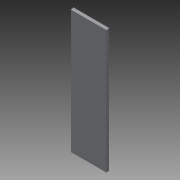
# Autodesk Inventor part: topback
Saved by Autodesk Inventor 2015 (Build 190159000, 159)
## iProperties
Created: 2015-02-03
Part Number: topback
Material: Generic
Document SubType Name: Modeling
Designer: rubidium
Density: 1 g/cm^3
Appearance: Default
Author: rubidium
Autodesk Inventor part; units mm, degrees
ref_plane "YZ Plane" through (0, 0, 0) normal (1, 0, 0) x (0, 1, 0)
ref_plane "XZ Plane" through (0, 0, 0) normal (0, 1, 0) x (-1, 0, 0)
ref_plane "XY Plane" through (0, 0, 0) normal (0, 0, 1) x (1, 0, 0)
sketch "Sketch1" plane through (0, 0, 0) normal (1, 0, 0) x (0, 1, 0)
  line L0 (879.2464, 0) -> (0, 0)
  line L1 (0, 0) -> (3.6409, -19.05)
  line L2 (3.6409, -19.05) -> (882.8804, -19.05)
  line L3 (882.8804, -19.05) -> (879.2464, 0)
  dimension "d0" = 879.2464
  dimension "d1" = 19.05
  dimension "d2" = 100.8
  dimension "d3" = 79.18
  constraints: 8 end point, 1 coincident, 1 horizontal, 1 parallel
  measures "d0" distance of L0.start L0.end
  measures "d1" distance between parallel lines of L2 L0
  measures "d2" angle of L3 L0
  measures "d3" angle of L0 L1
extrude "Extrusion1" add sketch "Sketch1" along normal blind 254
body "Solid1"
